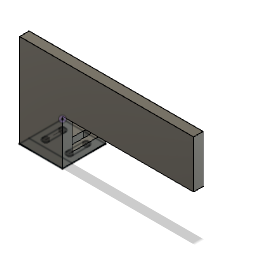
Nozzle Wipe - Left (Autodesk Fusion 360 design; units mm, degrees)
Autodesk Fusion 360 part; units mm, degrees
sketch "Skizze1" plane through (0, 0, 0) normal (0, 1, 0) x (1, 0, 0)
  line L0 (0, 0) -> (18, 0)
  line L1 (18, 0) -> (18, -18)
  line L2 (18, -18) -> (0, -18)
  line L3 (0, -18) -> (0, 0)
  line L4 (2.675, -4) -> (2.675, -11)
  arc A0 (2.675, -11) -> (5.325, -11) centre (4, -11) ccw
  line L5 (5.325, -11) -> (5.325, -4)
  arc A1 (5.325, -4) -> (2.675, -4) centre (4, -4) ccw
  line L6 (4, -4) -> (4, -11) construction
  line L7 (12.675, -4) -> (12.675, -11)
  arc A2 (12.675, -11) -> (15.325, -11) centre (14, -11) ccw
  line L8 (15.325, -11) -> (15.325, -4)
  arc A3 (15.325, -4) -> (12.675, -4) centre (14, -4) ccw
  line L9 (14, -4) -> (14, -11) construction
  line L10 (0, -14) -> (18, -14)
  dimension "d1" = 18
  dimension "d2" = 18
  dimension "d3" = 2.65
  dimension "d4" = 2.65
  dimension "d5" = 10
  dimension "d6" = 7
  dimension "d7" = 7
  dimension "d10" = 4
  dimension "d27" = 4
  dimension "d28" = 4
  constraint horizontal L0
  constraint vertical L1
  constraint horizontal L2
  constraint vertical L3
  constraint coincident L0.start L3.end
  constraint tangent L4 A0
  constraint tangent A0 L5
  constraint parallel L4 L5
  constraint tangent L5 A1
  constraint tangent L4 A1
  constraint vertical L6
  constraint tangent L7 A2
  constraint tangent A2 L8
  constraint parallel L7 L8
  constraint tangent L8 A3
  constraint tangent L7 A3
  constraint perpendicular L0 L9
  constraint horizontal A1.centre A3.centre
  constraint coincident L3 L10.start
  constraint coincident L1 L10.end
  constraint perpendicular L1 L10
  measures "d1" distance of L0.start L0.end
  measures "d2" distance of L0.start L2.end
  measures "d3" diameter of A0
  measures "d4" diameter of A2
  measures "d5" horizontal distance of A0.centre A2.centre
  measures "d6" distance of A1.centre A0.centre
  measures "d7" distance of A3.centre A2.centre
  measures "d10" distance of L1 A2.centre
  measures "d27" distance of L0 A1.centre
  measures "d28" distance of L2 L10
extrude "Extrusion1" add sketch "Skizze1" along normal blind 4
extrude "Extrusion2" add sketch "Skizze1" along normal blind 35 from surface at 4 contours L1 L2 L3 L10
sketch "Skizze2" plane through (18, 0, 0) normal (1, 0, 0) x (0, 0, -1)
  line L0 (-18, 0) -> (0, 0)
  line L1 (-16, 49) -> (-18, 49)
  line L2 (-18, 49) -> (-18, 0)
  line L3 (-14, 39) -> (-18, 39)
  line L4 (-18, 39) -> (-18, 19)
  line L5 (-18, 19) -> (-14, 19)
  line L6 (-14, 19) -> (-14, 39)
  line L7 (0, 0) -> (0, 4)
  line L8 (0, 4) -> (-16, 4)
  line L9 (-16, 4) -> (-16, 49)
  line L10 (-18, 0) -> (0, 0)
  line L11 (0, 0) -> (0, 4)
  line L12 (0, 4) -> (-14, 4)
  line L13 (-14, 4) -> (-14, 39)
  line L14 (-14, 39) -> (-18, 39)
  line L15 (-18, 39) -> (-18, 0)
  dimension "d17" = 20
  constraint horizontal L3
  constraint vertical L4
  constraint horizontal L5
  constraint vertical L6
  constraint coincident L4.end L15
  constraint coincident L3 L6.end
  constraint coincident L6 L3.start
  measures "d17" distance of L3.start L5.end
extrude "Extrusion3" add sketch "Skizze2" along normal blind 55 contours L2 L3 L4 L5 L9 L14 L15 | L3 L5 L6 L9 L13 L14
named bodies: "Nozzle Wipe - Left"
